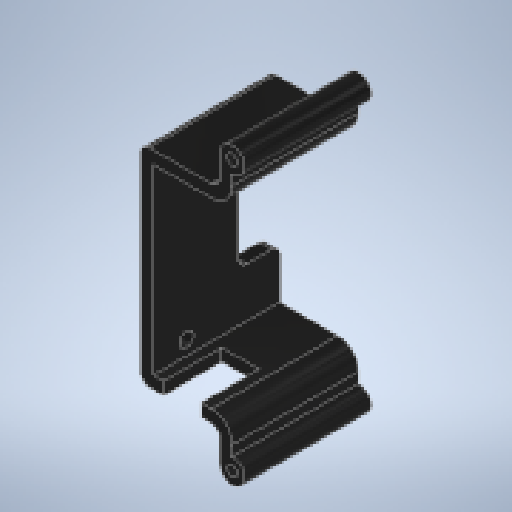
# Autodesk Inventor part: mune_2
Saved by Autodesk Inventor 2025.1 (Build 291241000, 241)
## iProperties
Created: 2024-09-03
Part Number: mune_2
Material: ABS プラスチック
Document SubType Name: Modeling
Designer: right
Density: 1.06 g/cm^3
Appearance: 滑らか - 黒
Mass: 9.57306 g
Surface Area: 73.943 cm^2
Volume: 9.03119 cm^3
Author: right
Autodesk Inventor part; units mm, degrees
ref_plane "YZ Plane" through (0, 0, 0) normal (1, 0, 0) x (0, 1, 0)
ref_plane "XZ Plane" through (0, 0, 0) normal (0, 1, 0) x (-1, 0, 0)
sketch "スケッチ1" plane through (0, 0, 0) normal (0, 0, 1) x (1, 0, 0)
  circle A0 centre (-7.5, -32.5) radius 1.6 projected
  circle A1 centre (-7.5, 32.5) radius 1.6 projected
  circle A2 centre (-7.5, -32.5) radius 1.3
  circle A3 centre (-7.5, 32.5) radius 1.3
  circle A4 centre (-7.5, 32.5) radius 3
  circle A5 centre (-7.5, -32.5) radius 3
  circle A6 centre (-7.5, 32.5) radius 1.6 projected
  circle A7 centre (7.5, -32.5) radius 1.6 projected
  circle A8 centre (7.5, 32.5) radius 1.6 projected
  circle A9 centre (-7.5, -32.5) radius 1.6 projected
  circle A10 centre (15.5, 0) radius 1.1 projected
  circle A11 centre (10.5, -5) radius 1.1 projected
  circle A12 centre (5.5, 0) radius 1.1 projected
  circle A13 centre (10.5, 5) radius 1.1 projected
  arc A14 (-10.5, -38) -> (-8.5, -40) centre (-8.5, -38) ccw projected
  line L0 (-8.5, -40) -> (8.5, -40) projected
  arc A15 (8.5, -40) -> (10.5, -38) centre (8.5, -38) ccw projected
  line L1 (10.5, -38) -> (10.5, -27) projected
  arc A16 (12.5, -25) -> (10.5, -27) centre (12.5, -27) ccw projected
  line L2 (12.5, -25) -> (18.5, -25) projected
  arc A17 (18.5, -25) -> (20.5, -23) centre (18.5, -23) ccw projected
  line L3 (20.5, -23) -> (20.5, 23) projected
  arc A18 (20.5, 23) -> (18.5, 25) centre (18.5, 23) ccw projected
  line L4 (18.5, 25) -> (12.5, 25) projected
  arc A19 (10.5, 27) -> (12.5, 25) centre (12.5, 27) ccw projected
  line L5 (10.5, 27) -> (10.5, 38) projected
  arc A20 (10.5, 38) -> (8.5, 40) centre (8.5, 38) ccw projected
  line L6 (8.5, 40) -> (-8.5, 40) projected
  arc A21 (-8.5, 40) -> (-10.5, 38) centre (-8.5, 38) ccw projected
  line L7 (-10.5, 38) -> (-10.5, 27) projected
  arc A22 (-12.5, 25) -> (-10.5, 27) centre (-12.5, 27) ccw projected
  line L8 (-12.5, 25) -> (-27.5, 25) projected
  arc A23 (-27.5, 25) -> (-29.5, 23) centre (-27.5, 23) ccw projected
  line L9 (-29.5, 23) -> (-29.5, -23) projected
  arc A24 (-29.5, -23) -> (-27.5, -25) centre (-27.5, -23) ccw projected
  line L10 (-27.5, -25) -> (-12.5, -25) projected
  arc A25 (-10.5, -27) -> (-12.5, -25) centre (-12.5, -27) ccw projected
  line L11 (-10.5, -27) -> (-10.5, -38) projected
  circle A26 centre (-8, 38) radius 1.1 projected
  circle A27 centre (-8, -38) radius 1.1 projected
  circle A28 centre (8, -38) radius 1.1 projected
  circle A29 centre (8, 38) radius 1.1 projected
  line L12 (-12.5, -22) -> (-26.5, -22)
  line L13 (-26.5, -22) -> (-26.5, 22)
  line L14 (-26.5, 22) -> (-12.5, 22)
  arc A30 (-12.5, 22) -> (-7.5, 27) centre (-12.5, 27) ccw
  line L15 (-7.5, 27) -> (-7.5, 37)
  line L16 (-7.5, 37) -> (7.5, 37)
  line L17 (7.5, 37) -> (7.5, 27)
  arc A31 (7.5, 27) -> (12.5, 22) centre (12.5, 27) ccw
  line L18 (12.5, 22) -> (17.5, 22)
  line L19 (17.5, 22) -> (17.5, -22)
  line L20 (17.5, -22) -> (12.5, -22)
  arc A32 (12.5, -22) -> (7.5, -27) centre (12.5, -27) ccw
  line L21 (7.5, -27) -> (7.5, -37)
  line L22 (7.5, -37) -> (-7.5, -37)
  line L23 (-7.5, -37) -> (-7.5, -27)
  arc A33 (-7.5, -27) -> (-12.5, -22) centre (-12.5, -27) ccw
  point P0 (0, 0)
  point P1 (-7.5, 29.5)
  point P2 (-10.5, 32.5)
  point P3 (-10.5, -32.5)
  point P4 (-7.5, -29.5)
  dimension "d0" = 2.6
  dimension "d1" = 2.6
  dimension "d2" = 6
  dimension "d3" = 6
  dimension "d4" = 3
  constraints: 24 end point, 8 centre point, 8 point on circle, 4 coincident, 15 other
  measures "d0" diameter of A2
  measures "d1" diameter of A3
  measures "d2" diameter of A4
  measures "d3" diameter of A5
  measures "d4" distance between parallel lines of L10 L12
ref_plane "作業平面1" through (-29.5, -40, 30.5) normal (0, 0, -1) x (0, 1, 0)
extrude "押し出し1" add sketch "スケッチ1" along normal up to surface (30.5 mm away) contours A0 L23 A2 | A0 L23 A5 | L23 A2 A0 | A0 L23 A5 | A5 L11 A25 L10 A24 L9 A23 L8 A22 L7 A4 L15 A30 L14 L13 L12 A33 L23 | L15 A1 A4 | A4 L15 A1 | L15 A3 A1 | A1 L15 A3
sketch "スケッチ2" plane through (-29.5, -23, 0) normal (-1, 0, 0) x (0, 0, 1)
  line L0 (0, 33) -> (10, 33)
  line L1 (10, 33) -> (10, 13)
  line L2 (10, 13) -> (0, 13)
  line L3 (0, 13) -> (0, 33)
  line L4 (0, 46) -> (0, 0) projected
  point P0 (0, 23)
  point P1 (10, 23)
  point P2 (0, 23)
  point P3 (0, 23)
  dimension "d7" = 10
  dimension "d8" = 20
  constraints: 8 end point, 4 midpoint, 2 parallel, 1 horizontal, 1 horizontal alignment, 1 perpendicular
  measures "d7" distance between parallel lines of L3 L1
  measures "d8" distance between parallel lines of L2 L0
extrude "押し出し2" cut sketch "スケッチ2" against normal through all
fillet "フィレット1" radius 2 4 edges at (-28, 10, 10) (-28, 10, 0) (-28, -10, 10) (-28, -10, 0)
sketch "スケッチ3" plane through (-27.5, -25, 0) normal (0, -1, 0) x (1, 0, 0)
  line L0 (15, 30.5) -> (1, 30.5) projected
  line L1 (3.5, 30.5) -> (12.5, 30.5)
  line L2 (12.5, 30.5) -> (12.5, 16.5)
  line L3 (12.5, 16.5) -> (3.5, 16.5)
  line L4 (3.5, 16.5) -> (3.5, 30.5)
  point P0 (27.5, 0)
  point P1 (8, 30.5)
  point P2 (8, 16.5)
  point P3 (12.5, 30.5)
  dimension "d12" = 9
  dimension "d13" = 14
  constraints: 8 end point, 2 midpoint, 2 parallel, 1 horizontal, 1 perpendicular, 1 point on line, 1 vertical alignment
  measures "d12" distance of L2.end L3.end
  measures "d13" distance of L1.end L2.end
extrude "押し出し3" cut sketch "スケッチ3" against normal up to surface (3 mm away)
sketch "スケッチ4" plane through (-29.5, -23, 30.5) normal (-1, 0, 0) x (0, 0, 1)
  circle A0 centre (-8, 41.5) radius 1.75
  circle A1 centre (-8, 4.5) radius 1.75
  line L0 (0, 46) -> (0, 0) projected
  point P0 (-30.5, 23)
  point P1 (0, 23)
  dimension "d16" = 3.5
  dimension "d17" = 3.5
  dimension "d18" = 37
  dimension "d19" = 18.5
  dimension "d20" = 8
  constraints: 2 centre point, 1 midpoint, 1 vertical alignment
  measures "d16" diameter of A0
  measures "d17" diameter of A1
  measures "d18" distance of A1.centre A0.centre
  measures "d19" vertical distance of point (0, 23) A0.centre
  measures "d20" distance from line of L0 A0.centre
extrude "押し出し4" cut sketch "スケッチ4" against normal through all
equation "\"d19\" = 0.5 * d18"
